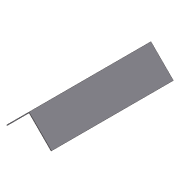
# Autodesk Inventor part: CornerSlider
Saved by Autodesk Inventor 2012 (Build 160160000, 160)
## iProperties
Created: 2013-01-06
Part Number: CornerSlider
Material: Aluminum-6061
Document SubType Name: Modeling
Designer: JesseK
Density: 2.71 g/cm^3
Mass: 1260.8 g
Surface Area: 2983.66 cm^2
Volume: 465.239 cm^3
Author: JesseK
Autodesk Inventor part; units mm, degrees
ref_plane "YZ Plane" through (0, 0, 0) normal (1, 0, 0) x (0, 1, 0)
ref_plane "XZ Plane" through (0, 0, 0) normal (0, 1, 0) x (-1, 0, 0)
ref_plane "XY Plane" through (0, 0, 0) normal (0, 0, 1) x (1, 0, 0)
sketch "Sketch1" plane through (0, 0, 0) normal (0, 0, 1) x (1, 0, 0)
  line L0 (0, 0) -> (-89.8026, -89.8026)
  line L1 (-89.8026, -89.8026) -> (-87.5575, -92.0476)
  line L2 (-87.5575, -92.0476) -> (0, -4.4901)
  line L3 (0, -4.4901) -> (87.5575, -92.0476)
  line L4 (87.5575, -92.0476) -> (89.8026, -89.8026)
  line L5 (89.8026, -89.8026) -> (0, 0)
  dimension "d0" = 3.175
  dimension "d1" = 127
  constraints: 12 end point, 4 parallel, 3 perpendicular
  measures "d0" distance of L0.end L1.end
  measures "d1" distance of L4.end L0.start
extrude "Extrusion1" add sketch "Sketch1" along normal blind 584.2
body "Solid1"
